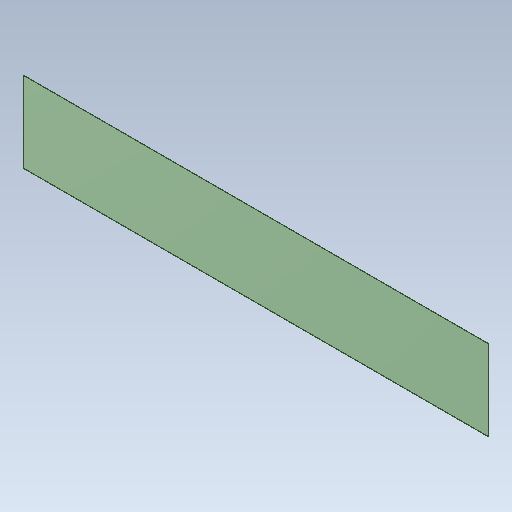
# Autodesk Inventor part: FTDI
Saved by Autodesk Inventor 2020 (Build 240168000, 168)
## iProperties
Created: 2019-05-24
Part Number: FTDI
Material: Generic
Document SubType Name: Modeling
Designer: psrob
Density: 1 g/cm^3
Appearance: 1X06, FTDI
Author: psrob
Autodesk Inventor part; units mm, degrees
ref_plane "YZ Plane" through (0, 0, 0) normal (1, 0, 0) x (0, 1, 0)
ref_plane "XZ Plane" through (0, 0, 0) normal (0, 1, 0) x (-1, 0, 0)
ref_plane "XY Plane" through (0, 0, 0) normal (0, 0, 1) x (1, 0, 0)
sketch "1X06, FTDI_30" plane through (0, 0, 0) normal (0, 0, 1) x (1, 0, 0)
  line L0 (-1.27, 1.3716) -> (13.97, 1.3716)
  line L1 (13.97, 1.3716) -> (13.97, -1.27)
  line L2 (13.97, -1.27) -> (-1.27, -1.27)
  line L3 (-1.27, -1.27) -> (-1.27, 1.3716)
  constraints: 8 end point
extrude "Extrusion1" add sketch "1X06, FTDI_30" along normal blind 0.01
body "Solid1"
